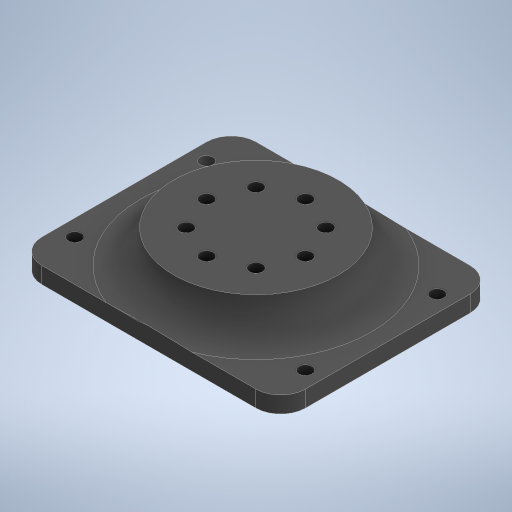
# Autodesk Inventor part: neck
Saved by Autodesk Inventor 2024.1 (Build 281209000, 209)
## iProperties
Created: 2024-10-11
Part Number: neck
Material: 一般
Document SubType Name: Modeling
Designer: hibik
Density: 1 g/cm^3
Appearance: 既定
Author: hibik
Autodesk Inventor part; units mm, degrees
ref_plane "YZ Plane" through (0, 0, 0) normal (1, 0, 0) x (0, 1, 0)
ref_plane "XZ Plane" through (0, 0, 0) normal (0, 1, 0) x (-1, 0, 0)
ref_plane "XY Plane" through (0, 0, 0) normal (0, 0, 1) x (1, 0, 0)
sketch "スケッチ1" plane through (0, 0, 0) normal (0, 1, 0) x (-1, 0, 0)
  line L0 (-16, -13) -> (16, -13)
  line L1 (16, -13) -> (16, 13)
  line L2 (16, 13) -> (-16, 13)
  line L3 (-16, 13) -> (-16, -13)
  line L4 (-16, -13) -> (16, 13) construction
  line L5 (16, -13) -> (-16, 13) construction
  line L6 (-14, -8) -> (14, -8) construction
  line L7 (14, -8) -> (14, 8)
  line L8 (14, 8) -> (-14, 8) construction
  line L9 (-14, 8) -> (-14, -8)
  line L10 (-14, -8) -> (14, 8) construction
  line L11 (14, -8) -> (-14, 8) construction
  circle A0 centre (14, -8) radius 0.8
  circle A1 centre (14, 8) radius 0.8
  circle A2 centre (-14, -8) radius 0.8
  circle A3 centre (-14, 8) radius 0.8
  point P0 (0, 0)
  dimension "d0" = 32
  dimension "d1" = 26
  dimension "d2" = 28
  dimension "d3" = 16
  dimension "d4" = 1.6
  dimension "d5" = 1.6
  dimension "d6" = 1.6
  dimension "d7" = 1.6
  constraints: 24 end point, 4 centre point, 4 coincident, 4 midpoint, 4 parallel, 2 horizontal, 2 perpendicular
  measures "d0" distance of L1.end L2.end
  measures "d1" distance of L0.end L1.end
  measures "d2" distance of L7.end L8.end
  measures "d3" distance of L6.end L7.end
  measures "d4" diameter of A0
  measures "d5" diameter of A1
  measures "d6" diameter of A2
  measures "d7" diameter of A3
extrude "押し出し1" add sketch "スケッチ1" along normal blind 2
sketch "スケッチ2" plane through (0, 2, 0) normal (0, 1, 0) x (1, 0, 0)
  circle A0 centre (0, 0) radius 6 construction
  circle A1 centre (0, 0) radius 10
  circle A2 centre (-6, 0) radius 0.8
  circle A3 centre (-4.2426, -4.2426) radius 0.8
  circle A4 centre (0, -6) radius 0.8
  circle A5 centre (4.2426, -4.2426) radius 0.8
  circle A6 centre (6, 0) radius 0.8
  circle A7 centre (4.2426, 4.2426) radius 0.8
  circle A8 centre (0, 6) radius 0.8
  circle A9 centre (-4.2426, 4.2426) radius 0.8
  dimension "d10" = 12
  dimension "d11" = 20
  dimension "d12" = 1.6
  dimension "d15" = 360
  constraints: 9 centre point, 2 coincident, 2 horizontal alignment, 19 other
  measures "d11" diameter of A1
  measures "d12" diameter of A2
extrude "押し出し2" add sketch "スケッチ2" along normal blind 4
fillet "フィレット1" radius 4 1 edges at (-10, 2, 0)
fillet "フィレット2" radius 3 4 edges at (16, 1, 13) (16, 1, -13) (-16, 1, 13) (-16, 1, -13)
